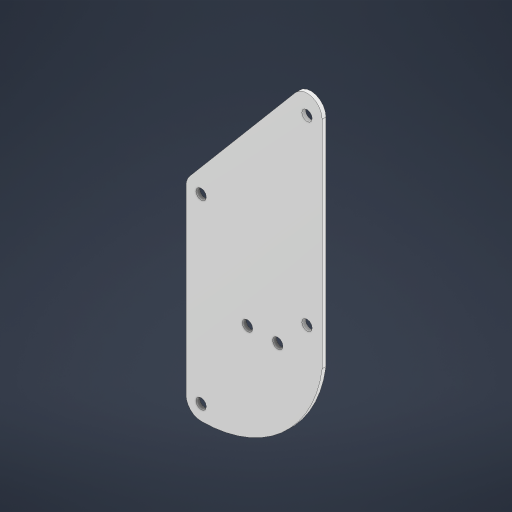
# Autodesk Inventor part: sled
Saved by Autodesk Inventor 2024 (Build 280153000, 153)
## iProperties
Created: 2023-10-18
Part Number: sled
Material: Acetal Resin, White
Document SubType Name: Sheet Metal
Designer: Averey Ku
Density: 1.425 g/cm^3
Appearance: Smooth - White
Flat Pattern Width: 14.1545 cm
Flat Pattern Length: 5.715 cm
Flat Pattern Area: 80.893 cm^2
Sheet Metal Rule: Default_mm
Sheet Metal Width: 5.573 in
Sheet Metal Length: 2.250 in
Sheet Metal Area: 12.538 in^2
Author: Averey Ku
Autodesk Inventor part; units mm, degrees
ref_plane "YZ Plane" through (0, 0, 0) normal (1, 0, 0) x (0, 1, 0)
ref_plane "XZ Plane" through (0, 0, 0) normal (0, 1, 0) x (-1, 0, 0)
ref_plane "XY Plane" through (0, 0, 0) normal (0, 0, 1) x (1, 0, 0)
sketch "Sketch1" plane through (0, 0, 0) normal (0, 0, 1) x (1, 0, 0)
  circle A0 centre (23.6047, -79.133) radius 2.1844
  circle A1 centre (23.6047, -2.933) radius 2.1844
  circle A2 centre (43.0738, -41.033) radius 2.1844
  circle A3 centre (55.7738, -41.033) radius 2.1844
  arc A4 (18.7529, 1.1636) -> (17.2547, -2.933) centre (23.6047, -2.933) ccw
  arc A5 (17.2547, -79.133) -> (23.607, -85.483) centre (23.6047, -79.133) ccw
  arc A6 (23.607, -85.483) -> (74.4047, -41.033) centre (23.5887, -34.2111) ccw
  line L0 (18.7529, 1.1636) -> (63.2029, 53.8087)
  line L1 (63.2029, 53.8087) -> (18.7529, 1.1636)
  line L2 (63.2029, 53.8087) -> (18.7529, 1.1636)
  line L3 (74.4047, -41.033) -> (74.4047, 49.7121)
  arc A7 (74.4047, 49.7121) -> (63.2029, 53.8087) centre (68.0547, 49.7121) ccw
  line L4 (17.2547, -79.133) -> (17.2547, -2.933)
  circle A8 centre (68.0547, -28.333) radius 2.1844
  circle A9 centre (68.0547, 47.867) radius 2.1844
  dimension "d12" = 12.7
  dimension "d13" = 12.7
  dimension "d14" = 6.35
  dimension "d15" = 4.3688
  dimension "d16" = 4.3688
  constraints: 10 centre point, 10 end point, 8 point on circle, 8 tangent, 2 coincident, 1 vertical
  measures "d12" diameter of A4
  measures "d13" diameter of A5
  measures "d14" radius of A7
  measures "d15" diameter of A8
  measures "d16" diameter of A9
extrude "Extrusion1" add sketch "Sketch1" along normal blind 1.5875
equation "\"BendRadius\" = Thickness"
equation "\"BendReliefWidth\" = Thickness"
equation "\"BendReliefDepth\" = 0.5 * Thickness"
equation "\"CornerReliefSize\" = 4 * Thickness"
equation "\"MinimumRemnant\" = 2 * Thickness"
equation "\"TransitionRadius\" = BendRadius"
equation "\"JacobiRadiusSize\" = BendRadius"
equation "\"GapSize\" = Thickness"
equation "\"Thickness\" = 1.5875"
body "Solid1"
